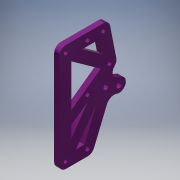
# Autodesk Inventor part: carriage plate square 2
Saved by Autodesk Inventor 2017 SP1 (Build 210196100, 196)
## iProperties
Created: 2018-01-19
Part Number: carriage plate square 2
Material: Aluminum 6061
Document SubType Name: Modeling
Designer: Ben
Density: 2.7 g/cm^3
Appearance: Smooth - Purple
Mass: 147.998 g
Surface Area: 209.147 cm^2
Volume: 54.8139 cm^3
Author: Ben
Autodesk Inventor part; units mm, degrees
ref_plane "YZ Plane" through (0, 0, 0) normal (1, 0, 0) x (0, 1, 0)
ref_plane "XZ Plane" through (0, 0, 0) normal (0, 1, 0) x (-1, 0, 0)
ref_plane "XY Plane" through (0, 0, 0) normal (0, 0, 1) x (1, 0, 0)
sketch "Sketch1" plane through (0, 0, 0) normal (1, 0, 0) x (0, 1, 0)
  line L0 (-420.7503, 12.7) -> (420.7488, 12.7) construction
  line L1 (420.7488, 12.7) -> (420.7488, -12.7) construction
  line L2 (420.7488, -12.7) -> (-420.7503, -12.7) construction
  line L3 (-420.7503, -12.7) -> (-420.7503, 12.7) construction
  line L4 (0, 0) -> (0, -26.6192) construction
  circle A0 centre (0, -26.6192) radius 2.54
  circle A1 centre (38.1, 26.6192) radius 2.54
  circle A2 centre (-76.2, 26.6192) radius 2.54
  line L5 (38.1, 26.6192) -> (-76.2, 26.6192) construction
  line L6 (0, 0) -> (0, 26.6192) construction
  circle A3 centre (0, -26.6192) radius 15.875 construction
  circle A4 centre (38.1, 26.6192) radius 15.875 construction
  circle A5 centre (-76.2, 26.6192) radius 15.875 construction
  line L7 (0, -26.6192) -> (-76.2, 26.6192) construction
  arc A6 (46.1645, 26.6192) -> (38.1, 34.6837) centre (38.1, 26.6192) ccw
  arc A7 (-76.2, 34.6837) -> (-84.2645, 26.6192) centre (-76.2, 26.6192) ccw
  line L8 (38.1, 34.6837) -> (-76.2, 34.6837)
  line L9 (46.1645, 26.6192) -> (46.1645, -19.05)
  line L10 (-84.2645, 0) -> (-84.2645, 26.6192)
  line L11 (-76.2, 26.6192) -> (-76.2, 0) construction
  line L12 (38.1, 26.6192) -> (38.1, 0) construction
  circle A8 centre (38.1, 0) radius 2.4892
  circle A9 centre (-76.2, 0) radius 2.4892
  line L13 (46.1645, 0) -> (-84.2645, 0) construction
  line L14 (-84.2645, 0) -> (-420.7503, 0) construction
  circle A10 centre (-19.05, 0) radius 2.4892
  line L15 (0, -26.6192) -> (38.1, 26.6192) construction
  line L16 (0, -26.6192) -> (0, -52.0192) construction
  line L17 (13.9446, -26.6192) -> (-16.4809, -26.6192) construction
  circle A11 centre (38.1, -19.05) radius 2.54
  circle A12 centre (-22.225, -22.225) radius 2.54
  line L18 (38.1, -19.05) -> (38.1, 0) construction
  arc A13 (39.6714, -26.9599) -> (46.1645, -19.05) centre (38.1, -19.05) ccw
  arc A14 (-84.2645, 0) -> (-79.2706, -7.4571) centre (-76.2, 0) ccw
  circle A15 centre (-28.575, -38.1) radius 3.302
  circle A16 centre (-28.575, -38.1) radius 9.525 construction
  line L19 (-28.575, -12.7) -> (-28.575, -28.575) construction
  line L20 (-28.575, -47.625) -> (133.2586, -47.625) construction
  line L21 (-28.575, -47.625) -> (-28.575, -47.625) construction
  arc A17 (-36.1151, -35.2394) -> (-41.3941, -23.0532) centre (-45.0208, -31.8608) ccw
  line L22 (-41.3941, -23.0532) -> (-79.2706, -7.4571)
  circle A18 centre (-28.575, -38.1) radius 14.2875 construction
  arc A19 (-5.6194, -32.4036) -> (1.5714, -34.5291) centre (0, -26.6192) ccw
  line L23 (-28.575, -38.1) -> (-22.225, -22.225) construction
  line L24 (-76.2, 0) -> (-22.225, -22.225) construction
  line L25 (1.5714, -34.5291) -> (39.6714, -26.9599)
  arc A20 (-36.1151, -35.2394) -> (-21.0873, -41.0951) centre (-28.575, -38.1) ccw
  circle A21 centre (38.1, 26.6192) radius 3.302 construction
  line L26 (-21.0873, -41.0951) -> (-18.7264, -35.1929)
  arc A22 (-5.6194, -32.4036) -> (-18.7264, -35.1929) centre (-11.2387, -38.1879) ccw
  point P0 (0, -42.4942)
  dimension "d3" = 31.75
  dimension "d0" = 25.4
  dimension "d1" = 5.08
  dimension "d2" = 13.9192
  dimension "d4" = 38.1
  dimension "d5" = 76.2
  dimension "d9" = 4.9784
  dimension "d10" = 25.4
  dimension "d14" = 6.35
  dimension "d15" = 9.525
  dimension "d17" = 3.175
  dimension "d18" = 22.225
  dimension "d19" = 6.604
  dimension "d26" = 19.05
  dimension "d28" = 0
  dimension "d31" = 28.575
  dimension "d34" = 34.925
  dimension "d35" = 28.575
  dimension "d37" = 4.7625
  dimension "d38" = 6.604
  dimension "d39" = 4.7625
  constraints: 54 end point, 22 centre point, 18 point on circle, 16 coincident, 14 tangent, 10 equal radius, 10 point on line, 8 vertical, 5 horizontal, 4 parallel, 4 perpendicular, 2 collinear, 2 midpoint, 1 vertical alignment, 4 other
  measures "d0" distance of L0.end L1.end
  measures "d1" diameter of A0
  measures "d2" distance from line of L2 L4.end
  measures "d4" horizontal distance of L5.start L4.end
  measures "d5" distance from line of A2.centre L6
  measures "d9" diameter of A8
  measures "d10" distance of L15.start L16.end
  measures "d14" distance from line of L2 L18.start
  measures "d15" distance from line of L2 L23.end
  measures "d17" vertical distance of L23.end L18.start
  measures "d18" horizontal distance of L23.end L4.end
  measures "d19" diameter of A15
  measures "d26" diameter of A16
  measures "d28" distance of L20.start L21.end
  measures "d31" distance from line of L23.start L4
  measures "d34" distance from line of L2 L20.start
  measures "d35" diameter of A18
  measures "d37" radial gap between concentric circles of A20 A15
  measures "d38" diameter of A21
  measures "d39" radial gap between concentric circles of A21 A6
extrude "Extrusion1" add sketch "Sketch1" along normal blind 6.35
sketch "Sketch3" plane through (0, 0, 0) normal (-1, 0, 0) x (0, 0, 1)
  circle A0 centre (-38.1, -28.575) radius 3.302 construction
  circle A1 centre (-22.225, -22.225) radius 2.54 construction
  circle A2 centre (-19.05, 38.1) radius 2.54 construction
  circle A3 centre (26.6192, -76.2) radius 2.54 construction
  circle A4 centre (26.6192, 38.1) radius 2.54 construction
  circle A5 centre (-26.6192, 0) radius 2.54 construction
  circle A6 centre (0, -19.05) radius 2.4892 construction
  circle A7 centre (0, -76.2) radius 2.4892 construction
  circle A8 centre (0, 38.1) radius 2.4892 construction
  arc A9 (34.6837, 38.1) -> (26.6192, 46.1645) centre (26.6192, 38.1) ccw construction
  line L0 (-19.05, 46.1645) -> (26.6192, 46.1645) construction
  arc A10 (-19.05, 46.1645) -> (-26.9599, 39.6714) centre (-19.05, 38.1) ccw construction
  arc A11 (-23.0532, -41.3941) -> (-35.2394, -36.1151) centre (-31.8608, -45.0208) ccw construction
  line L1 (-7.4571, -79.2706) -> (-23.0532, -41.3941) construction
  arc A12 (-7.4571, -79.2706) -> (0, -84.2645) centre (0, -76.2) ccw construction
  line L2 (26.6192, -84.2645) -> (0, -84.2645) construction
  arc A13 (26.6192, -84.2645) -> (34.6837, -76.2) centre (26.6192, -76.2) ccw construction
  line L3 (34.6837, 38.1) -> (34.6837, -76.2) construction
  circle A14 centre (26.6192, 38.1) radius 2.54 construction
  circle A15 centre (-26.6192, 0) radius 2.54 construction
  line L4 (26.6192, 38.1) -> (-26.6192, 0) construction
  circle A16 centre (26.6192, -76.2) radius 2.54 construction
  line L5 (-26.6192, 0) -> (26.6192, -76.2) construction
  line L6 (26.6192, -76.2) -> (26.6192, 38.1) construction
  line L7 (-19.05, 38.1) -> (-26.6192, 0) construction
  line L8 (-19.05, 38.1) -> (26.6192, 38.1) construction
  line L9 (-13.8374, 31.75) -> (6.835, 31.75)
  line L10 (6.835, 31.75) -> (-17.2637, 14.5038)
  line L11 (-17.2637, 14.5038) -> (-13.8374, 31.75)
  line L12 (-26.6192, 0) -> (0, -19.05) construction
  line L13 (-34.5291, 1.5714) -> (-26.9599, 39.6714) projected
  arc A17 (-34.5291, 1.5714) -> (-32.4036, -5.6194) centre (-26.6192, 0) ccw projected
  arc A18 (-35.1929, -18.7264) -> (-32.4036, -5.6194) centre (-38.1879, -11.2387) ccw projected
  line L14 (-41.0951, -21.0873) -> (-35.1929, -18.7264) projected
  arc A19 (-41.0951, -21.0873) -> (-35.2394, -36.1151) centre (-38.1, -28.575) ccw projected
  line L15 (20.2692, -25.7471) -> (-15.708, 0)
  line L16 (-15.708, 0) -> (20.2692, 25.7471)
  line L17 (20.2692, 25.7471) -> (20.2692, -25.7471)
  line L18 (-3.5012, 31.75) -> (-3.5012, 38.1) construction
  line L19 (-5.2144, 23.1269) -> (-1.5188, 17.963) construction
  line L20 (-1.5188, 17.963) -> (2.1767, 12.7992) construction
  line L21 (-15.5506, 23.1269) -> (-21.7788, 24.3643) construction
  line L22 (-3.7563, -8.5532) -> (-7.4518, -13.7171) construction
  line L23 (20.2692, 0) -> (26.6192, 0) construction
  line L24 (-38.1, -28.575) -> (-22.225, -22.225) construction
  line L25 (-22.225, -22.225) -> (0, -19.05) construction
  line L26 (-22.225, -22.225) -> (0, -76.2) construction
  line L27 (-0.2154, -26.7044) -> (20.2692, -56.024)
  line L28 (20.2692, -56.024) -> (20.2692, -41.3642)
  line L29 (20.2692, -41.3642) -> (-0.2154, -26.7044)
  line L30 (20.2692, -48.6941) -> (26.6192, -48.6941) construction
  line L31 (10.0269, -41.3642) -> (4.8215, -45.001) construction
  line L32 (0, -19.05) -> (26.6192, -38.1) construction
  line L33 (10.0269, -34.0343) -> (13.7224, -28.8704) construction
  line L34 (26.6192, -76.2) -> (0, -76.2) construction
  line L35 (-10.3634, -34.3542) -> (4.2525, -69.85)
  line L36 (4.2525, -69.85) -> (14.4364, -69.85)
  line L37 (14.4364, -69.85) -> (-10.3634, -34.3542)
  line L38 (9.3445, -69.85) -> (9.3445, -76.2) construction
  line L39 (4.8215, -45.001) -> (-0.3839, -48.6379) construction
  line L40 (-3.0554, -52.1021) -> (-8.9271, -54.5199) construction
  point P0 (0, 0)
  dimension "d40" = 6.35
  constraints: 70 end point, 14 point on line, 11 equal length, 11 parallel, 11 perpendicular, 9 midpoint, 4 vertical, 3 horizontal, 1 collinear
  measures "d40" distance of L18.start L18.end
extrude "Extrusion2" cut sketch "Sketch3" against normal through all
chamfer "Chamfer1" distance 3.175 angle 45 3 edges at (0, 35.6108, 0) (0, -21.5392, 0) (0, -78.6892, 0)
body "Solid1"
